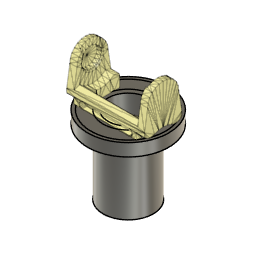
bed_chain (Autodesk Fusion 360 design; units mm, degrees)
Autodesk Fusion 360 part; units mm, degrees
sketch "Sketch1" plane through (0, 0, 0) normal (0, 0, 1) x (1, 0, 0)
  circle A0 centre (0, 0) radius 8.05
  circle A1 centre (0, 0) radius 6.5
  line L0 (1.8261, 6.2382) -> (1.8261, 7.8402)
  line L1 (-1.8261, 6.2382) -> (-1.8261, 7.8402)
  circle A2 centre (0, 0) radius 12
  circle A3 centre (0, 0) radius 13
  line L2 (1.8261, 7.8402) -> (1.8261, 12.8711)
  line L3 (-1.8261, 7.8402) -> (-1.8261, 12.8711)
  dimension "d1" = 16.1
  dimension "d2" = 13
  dimension "d5" = 24
  dimension "d6" = 26
  dimension "d15" = 3.95
  constraint coincident A0.centre A1.centre
  constraint concentric A0 A1
  constraint coincident A1 L0.start
  constraint coincident A0 L0.end
  constraint vertical L0
  constraint coincident A1 L1.start
  constraint coincident A0 L1.end
  constraint parallel L0 L1
  constraint concentric A1 A2
  constraint concentric A1 A3
  constraint coincident A3 L2.end
  constraint vertical L2
  constraint coincident A3 L3.end
  constraint parallel L1 L3
  measures "d1" diameter of A0
  measures "d2" diameter of A1
  measures "d5" diameter of A2
  measures "d6" diameter of A3
  measures "d15" distance of A0 A2
extrude "Extrude1" add sketch "Sketch1" along normal blind 25 contours A0 A1 L0 L1 picked at (-2.2084, 7.1864) makes body 1
other "Base Mesh Feature1"
other "Modify1"
extrude "Extrude2" add sketch "Sketch1" along normal blind 21 and the other way blind -25 separate body contours A2 A3 L2 L3 picked at (-2.4499, 12.3982) makes body 2
other "MeshPlaneCut1"
extrude "Extrude3" add sketch "Sketch1" along normal blind 25 and the other way blind -23 separate body contours A0 A2 L2 L3 picked at (-2.3989, 10.3883) makes body 3
